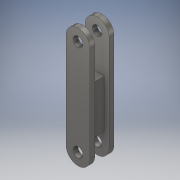
# Autodesk Inventor part: Crank
Saved by Autodesk Inventor 2019 (Build 230136000, 136)
## iProperties
Created: 2019-08-25
Part Number: Crank
Material: Steel, Mild
Document SubType Name: Modeling
Designer: DIBYOJYOTI
Density: 7.85 g/cm^3
Appearance: Semi-Polished
Mass: 19.8591 g
Surface Area: 24.299 cm^2
Volume: 2.52982 cm^3
Author: DIBYOJYOTI
Autodesk Inventor part; units mm, degrees
ref_plane "YZ Plane" through (0, 0, 0) normal (1, 0, 0) x (0, 1, 0)
ref_plane "XZ Plane" through (0, 0, 0) normal (0, 1, 0) x (-1, 0, 0)
ref_plane "XY Plane" through (0, 0, 0) normal (0, 0, 1) x (1, 0, 0)
sketch "Sketch1" plane through (0, 0, 0) normal (0, 0, 1) x (1, 0, 0)
  circle A0 centre (0, 0) radius 2.05
  arc A1 (-5, 0) -> (5, 0) centre (0, 0) ccw
  circle A2 centre (0, 40) radius 2.025
  arc A3 (5, 40) -> (-5, 40) centre (0, 40) ccw
  line L0 (-5, 40) -> (-5, 0)
  line L1 (5, 40) -> (5, 0)
  line L2 (0, 0) -> (0, 2.05)
  line L3 (0, 37.975) -> (0, 40)
  dimension "d0" = 4.1
  dimension "d3" = 4.05
  dimension "d1" = 10
  dimension "d2" = 40
  dimension "d4" = 10
  constraints: 8 end point, 4 coincident, 4 point on circle, 3 vertical, 2 centre point, 2 vertical alignment, 1 parallel, 4 other
  measures "d1" diameter of A1
  measures "d2" distance of L2.start L3.end
  measures "d4" diameter of A3
extrude "Extrusion1" add sketch "Sketch1" along normal blind 10
shell "Shell1" thickness 2 removed faces 4 at (3.9972, 43.0037, 6.6667) at (-4.9838, -0.4023, 6.6667) at (-5, 13.3333, 3.3333) at (5, 26.6667, 3.3333)
sketch "Sketch2" plane through (0, 40, 8) normal (0, 0, -1) x (-1, 0, 0)
  line L0 (-3, -35) -> (3, -35)
  line L1 (3, -35) -> (3, -15)
  line L2 (3, -15) -> (-3, -15)
  line L3 (-3, -15) -> (-3, -35)
  circle A0 centre (0, 0) radius 2.025 projected
  point P0 (0, -40)
  dimension "d13" = 6
  dimension "d14" = 20
  dimension "d18" = 5
  constraints: 8 end point, 2 parallel, 1 horizontal, 1 perpendicular
  measures "d13" distance of L2.end L1.end
  measures "d14" distance of L1.end L0.end
  measures "d18" distance from line of point (0, -40) L0
extrude "Extrusion2" add sketch "Sketch2" along normal blind 6 contours L3 L2 L1 L0
delete faces "Delete Face1" heal yes whole lump no faces at (4.0369, 0.3259, 4)
delete faces "Delete Face2" heal yes whole lump no faces at (4.0119, 40.3239, 4)
body "Solid1"
